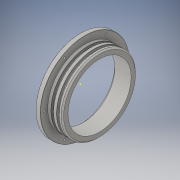
# Autodesk Inventor part: Oring Fitting Dome V1 end part
Saved by Autodesk Inventor 2016 (Build 200138000, 138)
## iProperties
Created: 2017-03-06
Part Number: Oring Fitting Dome V1 end part
Material: Generic
Document SubType Name: Modeling
Designer: Student
Density: 1 g/cm^3
Appearance: Default
Author: Student
Autodesk Inventor part; units mm, degrees
ref_plane "YZ Plane" through (0, 0, 0) normal (1, 0, 0) x (0, 1, 0)
ref_plane "XZ Plane" through (0, 0, 0) normal (0, 1, 0) x (-1, 0, 0)
ref_plane "XY Plane" through (0, 0, 0) normal (0, 0, 1) x (1, 0, 0)
sketch "Sketch1" plane through (0, 0, 0) normal (0, 1, 0) x (-1, 0, 0)
  line L0 (0, 0) -> (4.445, 0)
  line L1 (0, 0) -> (0, -3.175)
  line L2 (0, -3.175) -> (-3.175, -3.175)
  line L3 (-3.175, -3.175) -> (-3.175, 0)
  line L4 (-3.175, 0) -> (-7.62, 0)
  line L5 (-7.62, 0) -> (-7.62, -3.175)
  line L6 (-7.62, -3.175) -> (-10.795, -3.175)
  line L7 (-10.795, -3.175) -> (-10.795, 0)
  line L8 (-10.795, 0) -> (-15.24, 0)
  line L9 (-15.24, 0) -> (-15.24, -7.62)
  line L10 (-15.24, -7.62) -> (4.445, -7.62)
  line L11 (4.445, -7.62) -> (4.445, 0)
  line L12 (-15.24, 0) -> (-15.24, -50.292) construction
  line L13 (-15.24, -50.292) -> (-2.54, -50.292) construction
  dimension "d0" = 4.445
  dimension "d1" = 3.175
  dimension "d2" = 3.175
  dimension "d3" = 4.445
  dimension "d4" = 3.175
  dimension "d5" = 4.445
  dimension "d6" = 7.62
  dimension "d7" = 50.292
  dimension "d38" = 12.7
  constraints: 28 end point, 7 perpendicular, 4 point on line, 3 vertical, 2 horizontal, 1 collinear
  measures "d0" distance of L0.start L0.end
  measures "d1" distance of L0.start L1.end
  measures "d2" distance of L1.end L2.end
  measures "d3" distance of L3.end L4.end
  measures "d4" distance of L5.end L6.end
  measures "d5" distance of L7.end L8.end
  measures "d6" distance of L8.end L9.end
  measures "d7" distance of L8.end L12.end
  measures "d38" distance of L12.end L13.end
revolve "Revolution1" add sketch "Sketch1" angle 360 about axis through (15.24, 0, -50.292) along (-1, 0, 0)
sketch "Sketch2" plane through (-4.445, 0, -50.292) normal (-1, 0, 0) x (0, 0, 1)
  circle A0 centre (0, 0) radius 60.198
  circle A1 centre (0, 0) radius 42.672 projected
  dimension "d10" = 120.396
  constraints: 1 centre point, 1 coincident
  measures "d10" diameter of A0
extrude "Extrusion1" add sketch "Sketch2" along normal blind 6.096
sketch "Sketch3" plane through (-10.541, 0, -50.292) normal (-1, 0, 0) x (0, 0, 1)
  circle A0 centre (0, 0) radius 48.5013
  circle A1 centre (0, 0) radius 51.6763
  circle A2 centre (0, 0) radius 42.672 construction
  dimension "d42" = 3.175
  dimension "d62" = 97.0026
  constraints: 2 centre point, 2 coincident
  measures "d42" radial gap between concentric circles of A1 A0
  measures "d62" diameter of A0
extrude "Extrusion2" cut sketch "Sketch3" against normal blind 3.5306
chamfer "Chamfer1" distance 1.778 angle 45 1 edges at (15.24, 0, -100.584)
sketch "Sketch5" plane through (-10.541, 0, -50.292) normal (-1, 0, 0) x (0, 0, 1)
  circle A0 centre (0, 0) radius 55.245 construction
  circle A1 centre (0, 0) radius 42.672 projected
  circle A2 centre (0, 0) radius 48.5013 projected
  point P0 (-55.245, 0)
  point P1 (-27.6225, -47.8436)
  point P2 (27.6225, -47.8436)
  point P3 (55.245, 0)
  point P4 (27.6225, 47.8436)
  point P5 (-27.6225, 47.8436)
  dimension "d43" = 110.49
  dimension "d46" = 360
  constraints: 2 horizontal alignment, 10 other
hole "Hole1" at (-10.541, 0, -105.537) at (-10.541, -47.8436, -77.9145) at (-10.541, -47.8436, -22.6695) at (-10.541, 0, 4.953) at (-10.541, 47.8436, -22.6695) at (-10.541, 47.8436, -77.9145) direction (1, 0, 0) diameter 3 end through all
chamfer "Chamfer2" distance 0.254 angle 45 8 edges at (0, 0, -100.584) (3.175, 0, -100.584) (7.62, 0, -100.584) (10.795, 0, -100.584) (-10.541, 0, -101.9683) (-10.541, 0, -98.7933) (-10.541, 0, -110.49) (-4.445, 0, -110.49)
sketch "Sketch8" plane through (-10.541, 0, -50.292) normal (-1, 0, 0) x (0, 0, 1)
  circle A0 centre (0, 0) radius 48.2473 projected
  point P0 (50.292, 0)
chamfer "Chamfer3" distance 3.81 angle 45 1 edges at (-10.541, 0, -92.964)
sketch "Sketch9" plane through (-10.541, 0, -50.292) normal (-1, 0, 0) x (0, 0, 1)
  point P0 (50.292, 0)
body "Solid1"
